Autodesk Fusion 360 part; units mm, degrees
(part 2 of 3)
  line L1095 (-31.3966, -14.5) -> (-31.3966, -13.5)
  line L1096 (26.2931, -7) -> (27.2931, -7)
  line L1097 (-33.9483, -11) -> (-34.9483, -11)
  line L1098 (-31.3966, -11) -> (-32.3966, -11)
  line L1099 (-27.2931, -11) -> (-27.2931, -12)
  line L1100 (-28.8448, -12) -> (-28.8448, -11)
  line L1101 (-34.9483, -14.5) -> (-33.9483, -14.5)
  line L1102 (-33.9483, -13.5) -> (-34.9483, -13.5)
  line L1103 (-34.9483, -13.5) -> (-34.9483, -14.5)
  line L1104 (-31.5, -23) -> (-30.5, -23)
  line L1105 (-31.5, -21.5) -> (-31.5, -20.5)
  line L1106 (-30.5, -24) -> (-31.5, -24)
  line L1107 (-34, -23) -> (-33, -23)
  line L1108 (-28, -23) -> (-28, -24)
  line L1109 (-33, -20.5) -> (-33, -21.5)
  line L1110 (-36.5, -12) -> (-36.5, -11)
  line L1111 (22.1897, -3.5) -> (21.1897, -3.5)
  line L1112 (21.1897, -7) -> (22.1897, -7)
  line L1113 (-34.9483, -11) -> (-34.9483, -12)
  line L1114 (-29, -24) -> (-29, -23)
  line L1115 (-35.5, -23) -> (-35.5, -24)
  line L1116 (-36.5, -21.5) -> (-36.5, -20.5)
  line L1117 (-33.9483, -14.5) -> (-33.9483, -13.5)
  line L1118 (-29, -23) -> (-28, -23)
  line L1119 (-31.3966, -13.5) -> (-32.3966, -13.5)
  line L1120 (-36.5, -23) -> (-35.5, -23)
  line L1121 (-32.3966, -12) -> (-31.3966, -12)
  line L1122 (-33, -21.5) -> (-34, -21.5)
  line L1123 (-27.2931, -13.5) -> (-27.2931, -14.5)
  line L1124 (-29.8448, -12) -> (-28.8448, -12)
  line L1125 (-32.3966, -13.5) -> (-32.3966, -14.5)
  line L1126 (-37.5, -14.5) -> (-36.5, -14.5)
  line L1127 (-36.5, -20.5) -> (-35.5, -20.5)
  line L1128 (-36.5, -14.5) -> (-36.5, -13.5)
  line L1129 (-37.5, -11) -> (-37.5, -12)
  line L1130 (-29, -21.5) -> (-29, -20.5)
  line L1131 (-28.8448, -11) -> (-29.8448, -11)
  line L1132 (-34, -20.5) -> (-33, -20.5)
  line L1133 (-35.5, -20.5) -> (-35.5, -21.5)
  line L1134 (-33.9483, -12) -> (-33.9483, -11)
  line L1135 (-31.5, -24) -> (-31.5, -23)
  line L1136 (-33, -23) -> (-33, -24)
  line L1137 (-36.5, -13.5) -> (-37.5, -13.5)
  line L1138 (-29.8448, -14.5) -> (-28.8448, -14.5)
  line L1139 (36.5, -24) -> (35.5, -24)
  line L1140 (35.5, -20.5) -> (36.5, -20.5)
  line L1141 (36.5, -7) -> (37.5, -7)
  line L1142 (-6.8793, -11) -> (-6.8793, -12)
  line L1143 (-8.431, -12) -> (-8.431, -11)
  line L1144 (5.8793, -8.5) -> (5.8793, -9.5)
  line L1145 (4.3276, -9.5) -> (4.3276, -8.5)
  line L1146 (33.9483, -13.5) -> (33.9483, -14.5)
  line L1147 (3.3276, -8.5) -> (3.3276, -9.5)
  line L1148 (6.8793, -8.5) -> (5.8793, -8.5)
  line L1149 (3.3276, -11) -> (3.3276, -12)
  line L1150 (37.5, -7) -> (37.5, -6)
  line L1151 (1.7759, -8.5) -> (0.7759, -8.5)
  line L1152 (-5.8793, -7) -> (-5.8793, -6)
  line L1153 (-8.431, -3.5) -> (-9.431, -3.5)
  line L1154 (4.3276, -8.5) -> (3.3276, -8.5)
  line L1155 (36.5, -23) -> (35.5, -24) construction
  line L1156 (36.5, -6) -> (36.5, -7)
  line L1157 (5.8793, -12) -> (6.8793, -12)
  line L1158 (34, -23) -> (34, -24)
  line L1159 (0.7759, -9.5) -> (1.7759, -9.5)
  line L1160 (-9.431, -11) -> (-9.431, -12)
  line L1161 (37.5, -6) -> (36.5, -6)
  line L1162 (36.5, -21.5) -> (35.5, -21.5)
  line L1163 (-10.9828, -9.5) -> (-10.9828, -8.5)
  line L1164 (-9.431, -8.5) -> (-9.431, -9.5)
  line L1165 (33.9483, -3.5) -> (33.9483, -4.5)
  line L1166 (0.7759, -11) -> (0.7759, -12)
  line L1167 (-6.8793, -7) -> (-5.8793, -7)
  line L1168 (35.5, -21.5) -> (35.5, -20.5)
  line L1169 (36.5, -4.5) -> (37.5, -3.5) construction
  line L1170 (-5.8793, -4.5) -> (-5.8793, -3.5)
  line L1171 (33.9483, -11) -> (33.9483, -12)
  line L1172 (34.9483, -12) -> (34.9483, -11)
  line L1173 (36.5, -4.5) -> (37.5, -4.5)
  line L1174 (33.9483, -14.5) -> (34.9483, -14.5)
  line L1175 (-9.431, -9.5) -> (-8.431, -9.5)
  line L1176 (37.5, -13.5) -> (36.5, -13.5)
  line L1177 (-6.8793, -8.5) -> (-6.8793, -9.5)
  line L1178 (-8.431, -8.5) -> (-9.431, -8.5)
  line L1179 (-9.431, -12) -> (-8.431, -12)
  line L1180 (36.5, -3.5) -> (36.5, -4.5)
  line L1181 (3.3276, -6) -> (3.3276, -7)
  line L1182 (-9.431, -4.5) -> (-8.431, -4.5)
  line L1183 (-5.8793, -12) -> (-5.8793, -11)
  line L1184 (36.5, -13.5) -> (36.5, -14.5)
  line L1185 (1.7759, -12) -> (1.7759, -11)
  line L1186 (34.9483, -3.5) -> (33.9483, -3.5)
  line L1187 (37.5, -4.5) -> (36.5, -3.5) construction
  line L1188 (-6.8793, -9.5) -> (-5.8793, -9.5)
  line L1189 (-5.8793, -3.5) -> (-6.8793, -3.5)
  line L1190 (34.9483, -13.5) -> (33.9483, -13.5)
  line L1191 (1.7759, -6) -> (0.7759, -6)
  line L1192 (-5.8793, -8.5) -> (-6.8793, -8.5)
  line L1193 (34.9483, -11) -> (33.9483, -11)
  line L1194 (37.5, -3.5) -> (36.5, -3.5)
  line L1195 (37.5, -4.5) -> (37.5, -3.5)
  line L1196 (1.7759, -4.5) -> (1.7759, -3.5)
  line L1197 (36.5, -14.5) -> (37.5, -14.5)
  line L1198 (-8.431, -11) -> (-9.431, -11)
  line L1199 (34.9483, -14.5) -> (34.9483, -13.5)
  line L1200 (3.3276, -9.5) -> (4.3276, -9.5)
  line L1201 (33.9483, -4.5) -> (34.9483, -4.5)
  line L1202 (37.5, -14.5) -> (37.5, -13.5)
  line L1203 (-6.8793, -6) -> (-6.8793, -7)
  line L1204 (34.9483, -4.5) -> (34.9483, -3.5)
  line L1205 (17.5, -24) -> (17.5, -23)
  line L1206 (15, -23) -> (16, -23)
  line L1207 (12.5, -20.5) -> (13.5, -20.5)
  line L1208 (18.5, -23) -> (18.5, -24)
  line L1209 (17.5, -23) -> (18.5, -23)
  line L1210 (-10.9828, -8.5) -> (-11.9828, -8.5)
  line L1211 (-10.9828, -3.5) -> (-11.9828, -3.5)
  line L1212 (-11.9828, -7) -> (-10.9828, -7)
  line L1213 (13.5345, -8.5) -> (13.5345, -9.5)
  line L1214 (19.6379, -8.5) -> (18.6379, -8.5)
  line L1215 (-11.9828, -12) -> (-10.9828, -12)
  line L1216 (-11.9828, -4.5) -> (-10.9828, -4.5)
  line L1217 (-10.9828, -6) -> (-11.9828, -6)
  line L1218 (-11.9828, -14.5) -> (-10.9828, -14.5)
  line L1219 (-15, -24) -> (-16, -24)
  line L1220 (-15, -23) -> (-15, -24)
  line L1221 (15, -20.5) -> (16, -20.5)
  line L1222 (-13.5, -21.5) -> (-13.5, -20.5)
  line L1223 (-14.5345, -8.5) -> (-14.5345, -9.5)
  line L1224 (-11.9828, -6) -> (-11.9828, -7)
  line L1225 (-16.0862, -8.5) -> (-17.0862, -8.5)
  line L1226 (-17.0862, -14.5) -> (-16.0862, -14.5)
  line L1227 (14.5345, -14.5) -> (14.5345, -13.5)
  line L1228 (14.5345, -13.5) -> (13.5345, -13.5)
  line L1229 (19.6379, -14.5) -> (19.6379, -13.5)
  line L1230 (14.5345, -11) -> (13.5345, -11)
  line L1231 (17.0862, -12) -> (17.0862, -11)
  line L1232 (-16.0862, -3.5) -> (-17.0862, -3.5)
  line L1233 (-13.5345, -4.5) -> (-13.5345, -3.5)
  line L1234 (-13.5345, -14.5) -> (-13.5345, -13.5)
  line L1235 (13.5345, -12) -> (14.5345, -12)
  line L1236 (19.6379, -12) -> (19.6379, -11)
  line L1237 (-13.5345, -8.5) -> (-14.5345, -8.5)
  line L1238 (-14.5345, -9.5) -> (-13.5345, -9.5)
  line L1239 (-14.5345, -3.5) -> (-14.5345, -4.5)
  line L1240 (-14.5345, -6) -> (-14.5345, -7)
  line L1241 (14.5345, -12) -> (14.5345, -11)
  line L1242 (-14.5345, -14.5) -> (-13.5345, -14.5)
  line L1243 (17.0862, -13.5) -> (16.0862, -13.5)
  line L1244 (16.0862, -14.5) -> (17.0862, -14.5)
  line L1245 (-14.5345, -4.5) -> (-13.5345, -4.5)
  line L1246 (18.6379, -13.5) -> (18.6379, -14.5)
  line L1247 (-14.5345, -12) -> (-13.5345, -12)
  line L1248 (17.0862, -14.5) -> (17.0862, -13.5)
  line L1249 (-20, -20.5) -> (-20, -21.5)
  line L1250 (-27.2931, -14.5) -> (-26.2931, -14.5)
  line L1251 (-18.5, -21.5) -> (-18.5, -20.5)
  line L1252 (22.1897, -11) -> (21.1897, -11)
  line L1253 (19.6379, -9.5) -> (19.6379, -8.5)
  line L1254 (17.0862, -3.5) -> (16.0862, -3.5)
  line L1255 (14.5345, -7) -> (14.5345, -6)
  line L1256 (21, -23) -> (20, -24) construction
  line L1257 (-21, -24) -> (-21, -23)
  line L1258 (-17.5, -24) -> (-18.5, -24)
  line L1259 (-18.5, -20.5) -> (-17.5, -20.5)
  line L1260 (-18.5, -23) -> (-17.5, -23)
  line L1261 (18.6379, -7) -> (19.6379, -7)
  line L1262 (16.0862, -6) -> (16.0862, -7)
  line L1263 (14.5345, -3.5) -> (13.5345, -3.5)
  line L1264 (-26.5, -23) -> (-25.5, -24) construction
  line L1265 (13.5345, -9.5) -> (14.5345, -9.5)
  line L1266 (-16.0862, -6) -> (-17.0862, -6)
  line L1267 (-26.5, -23) -> (-25.5, -23)
  line L1268 (-20, -23) -> (-20, -24)
  line L1269 (18.6379, -4.5) -> (19.6379, -4.5)
  line L1270 (-25.5, -24) -> (-26.5, -24)
  line L1271 (-26.2931, -11) -> (-27.2931, -11)
  line L1272 (16.0862, -8.5) -> (16.0862, -9.5)
  line L1273 (-26.5, -24) -> (-26.5, -23)
  line L1274 (14.5345, -9.5) -> (14.5345, -8.5)
  line L1275 (-20, -24) -> (-21, -24)
  line L1276 (21, -24) -> (20, -24)
  line L1277 (-21, -23) -> (-20, -23)
  line L1278 (17.0862, -7) -> (17.0862, -6)
  line L1279 (13.5345, -6) -> (13.5345, -7)
  line L1280 (19.6379, -4.5) -> (19.6379, -3.5)
  line L1281 (17.0862, -9.5) -> (17.0862, -8.5)
  line L1282 (13.5345, -3.5) -> (13.5345, -4.5)
  line L1283 (14.5345, -8.5) -> (13.5345, -8.5)
  line L1284 (20, -23) -> (21, -24) construction
  line L1285 (-25.5, -23) -> (-25.5, -24)
  line L1286 (18.6379, -9.5) -> (19.6379, -9.5)
  line L1287 (16.0862, -3.5) -> (16.0862, -4.5)
  line L1288 (-17.0862, -7) -> (-16.0862, -7)
  line L1289 (16.0862, -4.5) -> (17.0862, -4.5)
  line L1290 (-26.5, -21.5) -> (-26.5, -20.5)
  line L1291 (21, -21.5) -> (20, -21.5)
  line L1292 (16.0862, -9.5) -> (17.0862, -9.5)
  line L1293 (16.0862, -7) -> (17.0862, -7)
  line L1294 (17.0862, -6) -> (16.0862, -6)
  line L1295 (-16.0862, -13.5) -> (-17.0862, -13.5)
  line L1296 (19.6379, -6) -> (18.6379, -6)
  line L1297 (18.6379, -3.5) -> (18.6379, -4.5)
  line L1298 (-37.5, -7) -> (-36.5, -7)
  line L1299 (-33.9483, -9.5) -> (-33.9483, -8.5)
  line L1300 (-24.7414, -13.5) -> (-24.7414, -14.5)
  line L1301 (-23.7414, -12) -> (-23.7414, -11)
  line L1302 (-28.8448, -4.5) -> (-28.8448, -3.5)
  line L1303 (-22.1897, -11) -> (-22.1897, -12)
  line L1304 (-18.6379, -7) -> (-18.6379, -6)
  line L1305 (-33.9483, -6) -> (-34.9483, -6)
  line L1306 (-26.2931, -13.5) -> (-27.2931, -13.5)
  line L1307 (-36.5, -6) -> (-37.5, -6)
  line L1308 (-19.6379, -12) -> (-18.6379, -12)
  line L1309 (-26.2931, -3.5) -> (-27.2931, -3.5)
  line L1310 (-27.2931, -6) -> (-27.2931, -7)
  line L1311 (23.7414, -11) -> (23.7414, -12)
  line L1312 (-21.1897, -4.5) -> (-21.1897, -3.5)
  line L1313 (21.1897, -3.5) -> (21.1897, -4.5)
  line L1314 (-28.8448, -6) -> (-29.8448, -6)
  line L1315 (-32.3966, -6) -> (-32.3966, -7)
  line L1316 (-23.7414, -8.5) -> (-24.7414, -8.5)
  line L1317 (-33.9483, -7) -> (-33.9483, -6)
  line L1318 (-34.9483, -4.5) -> (-33.9483, -4.5)
  line L1319 (-27.2931, -9.5) -> (-26.2931, -9.5)
  line L1320 (-26.2931, -9.5) -> (-26.2931, -8.5)
  line L1321 (-27.2931, -3.5) -> (-27.2931, -4.5)
  line L1322 (-31.3966, -7) -> (-31.3966, -6)
  line L1323 (23.7414, -8.5) -> (23.7414, -9.5)
  line L1324 (-24.7414, -8.5) -> (-24.7414, -9.5)
  line L1325 (-26.2931, -14.5) -> (-26.2931, -13.5)
  line L1326 (-22.1897, -13.5) -> (-22.1897, -14.5)
  line L1327 (27.2931, -3.5) -> (26.2931, -3.5)
  line L1328 (-34.9483, -9.5) -> (-33.9483, -9.5)
  line L1329 (-29.8448, -4.5) -> (-28.8448, -4.5)
  line L1330 (-18.6379, -12) -> (-18.6379, -11)
  line L1331 (-37.5, -6) -> (-37.5, -7)
  line L1332 (-24.7414, -9.5) -> (-23.7414, -9.5)
  line L1333 (-31.3966, -12) -> (-31.3966, -11)
  line L1334 (-26.2931, -6) -> (-27.2931, -6)
  line L1335 (-17.0862, -13.5) -> (-17.0862, -14.5)
  line L1336 (-22.1897, -14.5) -> (-21.1897, -14.5)
  line L1337 (-23.7414, -9.5) -> (-23.7414, -8.5)
  line L1338 (-37.5, -3.5) -> (-37.5, -4.5)
  line L1339 (-27.2931, -12) -> (-26.2931, -12)
  line L1340 (-18.6379, -8.5) -> (-19.6379, -8.5)
  line L1341 (-24.7414, -4.5) -> (-23.7414, -4.5)
  line L1342 (-19.6379, -7) -> (-18.6379, -7)
  line L1343 (-21.1897, -9.5) -> (-21.1897, -8.5)
  line L1344 (-21.1897, -8.5) -> (-22.1897, -8.5)
  line L1345 (-31.3966, -9.5) -> (-31.3966, -8.5)
  line L1346 (-37.5, -9.5) -> (-36.5, -9.5)
  line L1347 (27.2931, -7) -> (27.2931, -6)
  line L1348 (-23.7414, -3.5) -> (-24.7414, -3.5)
  line L1349 (-31.3966, -4.5) -> (-31.3966, -3.5)
  line L1350 (-18.6379, -6) -> (-19.6379, -6)
  line L1351 (-18.6379, -13.5) -> (-19.6379, -13.5)
  line L1352 (-33.9483, -8.5) -> (-34.9483, -8.5)
  line L1353 (-21.1897, -7) -> (-21.1897, -6)
  line L1354 (-37.5, -8.5) -> (-37.5, -9.5)
  line L1355 (-34.9483, -7) -> (-33.9483, -7)
  line L1356 (-22.1897, -12) -> (-21.1897, -12)
  line L1357 (-27.2931, -7) -> (-26.2931, -7)
  line L1358 (-29.8448, -11) -> (-29.8448, -12)
  line L1359 (-17.0862, -11) -> (-17.0862, -12)
  line L1360 (-24.7414, -14.5) -> (-23.7414, -14.5)
  line L1361 (22.1897, -7) -> (22.1897, -6)
  line L1362 (-32.3966, -14.5) -> (-31.3966, -14.5)
  line L1363 (-19.6379, -14.5) -> (-18.6379, -14.5)
  line L1364 (-37.5, -13.5) -> (-37.5, -14.5)
  line L1365 (-23.7414, -13.5) -> (-24.7414, -13.5)
  line L1366 (-33, -24) -> (-34, -24)
  line L1367 (-21.1897, -11) -> (-22.1897, -11)
  line L1368 (-27.2931, -8.5) -> (-27.2931, -9.5)
  line L1369 (-30.5, -21.5) -> (-31.5, -21.5)
  line L1370 (-24.7414, -7) -> (-23.7414, -7)
  line L1371 (23.7414, -3.5) -> (23.7414, -4.5)
  line L1372 (23.7414, -7) -> (24.7414, -7)
  line L1373 (26.2931, -3.5) -> (26.2931, -4.5)
  line L1374 (-26.2931, -12) -> (-26.2931, -11)
  line L1375 (21.1897, -4.5) -> (22.1897, -4.5)
  line L1376 (-21.1897, -12) -> (-21.1897, -11)
  line L1377 (-34, -21.5) -> (-34, -20.5)
  line L1378 (-28, -20.5) -> (-28, -21.5)
  line L1379 (-28, -24) -> (-29, -24)
  line L1380 (-29, -20.5) -> (-28, -20.5)
  line L1381 (24.7414, -7) -> (24.7414, -6)
  line L1382 (-27.2931, -4.5) -> (-26.2931, -4.5)
  line L1383 (-28.8448, -14.5) -> (-28.8448, -13.5)
  line L1384 (-35.5, -21.5) -> (-36.5, -21.5)
  line L1385 (-24.7414, -11) -> (-24.7414, -12)
  line L1386 (21.1897, -6) -> (21.1897, -7)
  line L1387 (-30.5, -23) -> (-30.5, -24)
  line L1388 (-23.7414, -11) -> (-24.7414, -11)
  line L1389 (26.2931, -4.5) -> (27.2931, -4.5)
  line L1390 (-19.6379, -11) -> (-19.6379, -12)
  line L1391 (-34, -24) -> (-34, -23)
  line L1392 (-23.7414, -4.5) -> (-23.7414, -3.5)
  line L1393 (-32.3966, -11) -> (-32.3966, -12)
  line L1394 (27.2931, -6) -> (26.2931, -6)
  line L1395 (-23.7414, -6) -> (-24.7414, -6)
  line L1396 (-21.1897, -14.5) -> (-21.1897, -13.5)
  line L1397 (24.7414, -4.5) -> (24.7414, -3.5)
  line L1398 (26.2931, -6) -> (26.2931, -7)
  line L1399 (22.1897, -4.5) -> (22.1897, -3.5)
  line L1400 (-23.7414, -14.5) -> (-23.7414, -13.5)
  line L1401 (-31.5, -20.5) -> (-30.5, -20.5)
  line L1402 (23.7414, -4.5) -> (24.7414, -4.5)
  line L1403 (23.7414, -6) -> (23.7414, -7)
  line L1404 (27.2931, -4.5) -> (27.2931, -3.5)
  line L1405 (22.1897, -6) -> (21.1897, -6)
  line L1406 (-24.7414, -12) -> (-23.7414, -12)
  line L1407 (-18.6379, -14.5) -> (-18.6379, -13.5)
  line L1408 (-35.5, -24) -> (-36.5, -24)
  line L1409 (-30.5, -20.5) -> (-30.5, -21.5)
  line L1410 (24.7414, -6) -> (23.7414, -6)
  line L1411 (-29.8448, -13.5) -> (-29.8448, -14.5)
  line L1412 (-34.9483, -12) -> (-33.9483, -12)
  line L1413 (-36.5, -24) -> (-36.5, -23)
  line L1414 (-16.0862, -12) -> (-16.0862, -11)
  line L1415 (20, -20.5) -> (21, -20.5)
  line L1416 (-11.9828, -11) -> (-11.9828, -12)
  line L1417 (-13.5345, -3.5) -> (-14.5345, -3.5)
  line L1418 (-16.0862, -4.5) -> (-16.0862, -3.5)
  line L1419 (-14.5345, -13.5) -> (-14.5345, -14.5)
  line L1420 (-13.5345, -12) -> (-13.5345, -11)
  line L1421 (-16.0862, -11) -> (-17.0862, -11)
  line L1422 (-13.5345, -7) -> (-13.5345, -6)
  line L1423 (13.5, -24) -> (12.5, -24)
  line L1424 (-13.5345, -11) -> (-14.5345, -11)
  line L1425 (-11.9828, -13.5) -> (-11.9828, -14.5)
  line L1426 (16.0862, -13.5) -> (16.0862, -14.5)
  line L1427 (18.6379, -14.5) -> (19.6379, -14.5)
  line L1428 (-16.0862, -9.5) -> (-16.0862, -8.5)
  line L1429 (13.5345, -14.5) -> (14.5345, -14.5)
  line L1430 (17.0862, -11) -> (16.0862, -11)
  line L1431 (-17.0862, -12) -> (-16.0862, -12)
  line L1432 (18.6379, -11) -> (18.6379, -12)
  line L1433 (18.6379, -8.5) -> (18.6379, -9.5)
  line L1434 (-18.6379, -9.5) -> (-18.6379, -8.5)
  line L1435 (-31.3966, -8.5) -> (-32.3966, -8.5)
  line L1436 (-32.3966, -9.5) -> (-31.3966, -9.5)
  line L1437 (23.7414, -9.5) -> (24.7414, -9.5)
  line L1438 (25.5, -21.5) -> (25.5, -20.5)
  line L1439 (21.1897, -13.5) -> (21.1897, -14.5)
  line L1440 (22.1897, -13.5) -> (21.1897, -13.5)
  line L1441 (-25.5, -23) -> (-26.5, -24) construction
  line L1442 (18.6379, -6) -> (18.6379, -7)
  line L1443 (-29.8448, -8.5) -> (-29.8448, -9.5)
  line L1444 (-20, -21.5) -> (-21, -21.5)
  line L1445 (26.2931, -9.5) -> (27.2931, -9.5)
  line L1446 (-17.5, -21.5) -> (-18.5, -21.5)
  line L1447 (-18.6379, -4.5) -> (-18.6379, -3.5)
  line L1448 (21.1897, -11) -> (21.1897, -12)
  line L1449 (24.7414, -12) -> (24.7414, -11)
  line L1450 (-31.3966, -6) -> (-32.3966, -6)
  line L1451 (-26.5, -20.5) -> (-25.5, -20.5)
  line L1452 (-17.5, -23) -> (-17.5, -24)
  line L1453 (-17.0862, -3.5) -> (-17.0862, -4.5)
  line L1454 (-19.6379, -6) -> (-19.6379, -7)
  line L1455 (27.2931, -9.5) -> (27.2931, -8.5)
  line L1456 (26.5, -23) -> (26.5, -24)
  line L1457 (-32.3966, -3.5) -> (-32.3966, -4.5)
  line L1458 (17.0862, -4.5) -> (17.0862, -3.5)
  line L1459 (-21, -20.5) -> (-20, -20.5)
  line L1460 (23.7414, -14.5) -> (24.7414, -14.5)
  line L1461 (24.7414, -8.5) -> (23.7414, -8.5)
  line L1462 (26.2931, -11) -> (26.2931, -12)
  line L1463 (14.5345, -6) -> (13.5345, -6)
  line L1464 (24.7414, -9.5) -> (24.7414, -8.5)
  line L1465 (-25.5, -21.5) -> (-26.5, -21.5)
  line L1466 (-22.1897, -4.5) -> (-21.1897, -4.5)
  line L1467 (14.5345, -4.5) -> (14.5345, -3.5)
  line L1468 (21, -20.5) -> (21, -21.5)
  line L1469 (24.7414, -14.5) -> (24.7414, -13.5)
  line L1470 (21.1897, -12) -> (22.1897, -12)
  line L1471 (13.5345, -4.5) -> (14.5345, -4.5)
  line L1472 (-25.5, -20.5) -> (-25.5, -21.5)
  line L1473 (22.1897, -9.5) -> (22.1897, -8.5)
  line L1474 (17.0862, -8.5) -> (16.0862, -8.5)
  line L1475 (19.6379, -7) -> (19.6379, -6)
  line L1476 (24.7414, -13.5) -> (23.7414, -13.5)
  line L1477 (21, -23) -> (21, -24)
  line L1478 (25.5, -20.5) -> (26.5, -20.5)
  line L1479 (-18.5, -24) -> (-18.5, -23)
  line L1480 (-22.1897, -9.5) -> (-21.1897, -9.5)
  line L1481 (13.5345, -7) -> (14.5345, -7)
  line L1482 (-31.3966, -3.5) -> (-32.3966, -3.5)
  line L1483 (21.1897, -9.5) -> (22.1897, -9.5)
  line L1484 (27.2931, -8.5) -> (26.2931, -8.5)
  line L1485 (27.2931, -13.5) -> (26.2931, -13.5)
  line L1486 (26.2931, -13.5) -> (26.2931, -14.5)
  line L1487 (-17.5, -20.5) -> (-17.5, -21.5)
  line L1488 (21.1897, -14.5) -> (22.1897, -14.5)
  line L1489 (-21, -21.5) -> (-21, -20.5)
  line L1490 (19.6379, -3.5) -> (18.6379, -3.5)
  line L1491 (-29.8448, -7) -> (-28.8448, -7)
  line L1492 (-19.6379, -4.5) -> (-18.6379, -4.5)
  line L1493 (27.2931, -14.5) -> (27.2931, -13.5)
  line L1494 (-19.6379, -9.5) -> (-18.6379, -9.5)
  line L1495 (-34.9483, -8.5) -> (-34.9483, -9.5)
  line L1496 (-28.8448, -8.5) -> (-29.8448, -8.5)
  line L1497 (-33.9483, -3.5) -> (-34.9483, -3.5)
  line L1498 (26.2931, -14.5) -> (27.2931, -14.5)
  line L1499 (-36.5, -4.5) -> (-36.5, -3.5)
  line L1500 (22.1897, -8.5) -> (21.1897, -8.5)
  line L1501 (-33.9483, -4.5) -> (-33.9483, -3.5)
  line L1502 (-19.6379, -3.5) -> (-19.6379, -4.5)
  line L1503 (-32.3966, -4.5) -> (-31.3966, -4.5)
  line L1504 (-36.5, -9.5) -> (-36.5, -8.5)
  line L1505 (-29.8448, -9.5) -> (-28.8448, -9.5)
  line L1506 (23.7414, -12) -> (24.7414, -12)
  line L1507 (-32.3966, -7) -> (-31.3966, -7)
  line L1508 (-34.9483, -3.5) -> (-34.9483, -4.5)
  line L1509 (-28.8448, -3.5) -> (-29.8448, -3.5)
  line L1510 (-23.7414, -7) -> (-23.7414, -6)
  line L1511 (22.1897, -12) -> (22.1897, -11)
  line L1512 (-21.1897, -6) -> (-22.1897, -6)
  line L1513 (-36.5, -7) -> (-36.5, -6)
  line L1514 (-18.6379, -3.5) -> (-19.6379, -3.5)
  line L1515 (-29.8448, -3.5) -> (-29.8448, -4.5)
  line L1516 (-32.3966, -8.5) -> (-32.3966, -9.5)
  line L1517 (27.2931, -12) -> (27.2931, -11)
  line L1518 (-36.5, -8.5) -> (-37.5, -8.5)
  line L1519 (21.1897, -8.5) -> (21.1897, -9.5)
  line L1520 (25.5, -24) -> (25.5, -23)
  line L1521 (-34.9483, -6) -> (-34.9483, -7)
  line L1522 (26.2931, -8.5) -> (26.2931, -9.5)
  line L1523 (26.2931, -12) -> (27.2931, -12)
  line L1524 (-26.2931, -4.5) -> (-26.2931, -3.5)
  line L1525 (-19.6379, -13.5) -> (-19.6379, -14.5)
  line L1526 (-19.6379, -8.5) -> (-19.6379, -9.5)
  line L1527 (-22.1897, -8.5) -> (-22.1897, -9.5)
  line L1528 (27.2931, -11) -> (26.2931, -11)
  line L1529 (25.5, -23) -> (26.5, -23)
  line L1530 (26.5, -21.5) -> (25.5, -21.5)
  line L1531 (-22.1897, -7) -> (-21.1897, -7)
  line L1532 (-26.2931, -8.5) -> (-27.2931, -8.5)
  line L1533 (-37.5, -4.5) -> (-36.5, -4.5)
  line L1534 (-17.0862, -6) -> (-17.0862, -7)
  line L1535 (26.5, -24) -> (25.5, -24)
  line L1536 (24.7414, -11) -> (23.7414, -11)
  line L1537 (-22.1897, -3.5) -> (-22.1897, -4.5)
  line L1538 (26.5, -20.5) -> (26.5, -21.5)
  line L1539 (-28.8448, -9.5) -> (-28.8448, -8.5)
  line L1540 (-24.7414, -6) -> (-24.7414, -7)
  line L1541 (23.7414, -13.5) -> (23.7414, -14.5)
  line L1542 (-17.0862, -8.5) -> (-17.0862, -9.5)
  line L1543 (-24.7414, -3.5) -> (-24.7414, -4.5)
  line L1544 (-22.1897, -6) -> (-22.1897, -7)
  line L1545 (-26.2931, -7) -> (-26.2931, -6)
  line L1546 (-18.6379, -11) -> (-19.6379, -11)
  line L1547 (-36.5, -3.5) -> (-37.5, -3.5)
  line L1548 (-21.1897, -13.5) -> (-22.1897, -13.5)
  line L1549 (22.1897, -14.5) -> (22.1897, -13.5)
  line L1550 (-28.8448, -7) -> (-28.8448, -6)
  line L1551 (-29.8448, -6) -> (-29.8448, -7)
  line L1552 (-21.1897, -3.5) -> (-22.1897, -3.5)
  line L1553 (28.8448, -7) -> (29.8448, -7)
  line L1554 (29.8448, -13.5) -> (28.8448, -13.5)
  line L1555 (28.8448, -13.5) -> (28.8448, -14.5)
  line L1556 (4.5, -23) -> (5.5, -24) construction
  line L1557 (29.8448, -7) -> (29.8448, -6)
  line L1558 (-6.8793, -13.5) -> (-6.8793, -14.5)
  line L1559 (29.8448, -14.5) -> (29.8448, -13.5)
  line L1560 (-8.431, -14.5) -> (-8.431, -13.5)
  line L1561 (3, -24) -> (2, -24)
  line L1562 (-9.431, -13.5) -> (-9.431, -14.5)
  line L1563 (6.8793, -14.5) -> (6.8793, -13.5)
  line L1564 (5.5, -23) -> (5.5, -24)
  line L1565 (29.8448, -6) -> (28.8448, -6)
  line L1566 (3, -20.5) -> (3, -21.5)
  line L1567 (-10.9828, -14.5) -> (-10.9828, -13.5)
  line L1568 (-10, -21.5) -> (-11, -21.5)
  line L1569 (3.3276, -14.5) -> (4.3276, -14.5)
  line L1570 (-0.7759, -11) -> (-1.7759, -11)
  line L1571 (-1.7759, -12) -> (-0.7759, -12)
  line L1572 (11.9828, -11) -> (10.9828, -11)
  line L1573 (-3.3276, -6) -> (-4.3276, -6)
  line L1574 (-0.7759, -13.5) -> (-1.7759, -13.5)
  line L1575 (8.431, -3.5) -> (8.431, -4.5)
  line L1576 (-0.7759, -14.5) -> (-0.7759, -13.5)
  line L1577 (8.431, -9.5) -> (9.431, -9.5)
  line L1578 (10.9828, -11) -> (10.9828, -12)
  line L1579 (-1.7759, -11) -> (-1.7759, -12)
  line L1580 (9.431, -11) -> (8.431, -11)
  line L1581 (-4.3276, -3.5) -> (-4.3276, -4.5)
  line L1582 (8.431, -7) -> (9.431, -7)
  line L1583 (-4.3276, -6) -> (-4.3276, -7)
  line L1584 (-3.3276, -7) -> (-3.3276, -6)
  line L1585 (-1.7759, -6) -> (-1.7759, -7)
  line L1586 (9.431, -7) -> (9.431, -6)
  line L1587 (-1.7759, -7) -> (-0.7759, -7)
  line L1588 (-3.3276, -3.5) -> (-4.3276, -3.5)
  line L1589 (10.9828, -7) -> (11.9828, -7)
  line L1590 (10.9828, -4.5) -> (11.9828, -4.5)
  line L1591 (-4.3276, -8.5) -> (-4.3276, -9.5)
  line L1592 (10.9828, -3.5) -> (10.9828, -4.5)
  line L1593 (11.9828, -8.5) -> (10.9828, -8.5)
  line L1594 (-3.3276, -8.5) -> (-4.3276, -8.5)
  line L1595 (11.9828, -7) -> (11.9828, -6)
  line L1596 (9.431, -4.5) -> (9.431, -3.5)
  line L1597 (-1.7759, -9.5) -> (-0.7759, -9.5)
  line L1598 (-1.7759, -8.5) -> (-1.7759, -9.5)
  line L1599 (9.431, -9.5) -> (9.431, -8.5)
  line L1600 (-1.7759, -3.5) -> (-1.7759, -4.5)
  line L1601 (10, -23) -> (11, -23)
  line L1602 (12.5, -21.5) -> (12.5, -20.5)
  line L1603 (-3, -21.5) -> (-3, -20.5)
  line L1604 (-2, -21.5) -> (-3, -21.5)
  line L1605 (11, -23) -> (11, -24)
  line L1606 (-2, -20.5) -> (-2, -21.5)
  line L1607 (-4.5, -23) -> (-4.5, -24)
  line L1608 (-0.5, -23) -> (0.5, -23)
  line L1609 (10, -20.5) -> (11, -20.5)
  line L1610 (10, -24) -> (10, -23)
  line L1611 (10.9828, -13.5) -> (10.9828, -14.5)
  line L1612 (9.431, -14.5) -> (9.431, -13.5)
  line L1613 (9.431, -13.5) -> (8.431, -13.5)
  line L1614 (11, -21.5) -> (10, -21.5)
  line L1615 (11.9828, -14.5) -> (11.9828, -13.5)
  line L1616 (-1.7759, -13.5) -> (-1.7759, -14.5)
  line L1617 (10.9828, -14.5) -> (11.9828, -14.5)
  line L1618 (-1.7759, -14.5) -> (-0.7759, -14.5)
  line L1619 (10, -21.5) -> (10, -20.5)
  line L1620 (-3.3276, -11) -> (-4.3276, -11)
  line L1621 (-3.3276, -13.5) -> (-4.3276, -13.5)
  line L1622 (8.431, -13.5) -> (8.431, -14.5)
  line L1623 (11, -24) -> (10, -24)
  line L1624 (8.431, -14.5) -> (9.431, -14.5)
  line L1625 (12.5, -24) -> (12.5, -23)
  line L1626 (-4.3276, -11) -> (-4.3276, -12)
  line L1627 (11, -20.5) -> (11, -21.5)
  line L1628 (-3.3276, -12) -> (-3.3276, -11)
  line L1629 (11.9828, -13.5) -> (10.9828, -13.5)
  line L1630 (-4.3276, -14.5) -> (-3.3276, -14.5)
  line L1631 (-3.3276, -14.5) -> (-3.3276, -13.5)
  line L1632 (-4.3276, -13.5) -> (-4.3276, -14.5)
  line L1633 (-4.3276, -12) -> (-3.3276, -12)
  line L1634 (-0.7759, -12) -> (-0.7759, -11)
  point P0 (36, 23.5)
  point P1 (20.5, 23.5)
  point P2 (5, 23.5)
  point P3 (-10.5, 23.5)
  point P4 (-26, 23.5)
  point P5 (37, 4)
  point P6 (36, -23.5)
  point P7 (37, -4)
  point P8 (-26, -23.5)
  point P9 (20.5, -23.5)
  point P10 (5, -23.5)
  point P11 (-10.5, -23.5)
  dimension "d12" = 2
  dimension "d14" = 1
  dimension "d15" = 3
  dimension "d16" = 5
  dimension "d23" = 1
  dimension "d27" = -10
  dimension "d31" = -62
  dimension "d32" = 0
  dimension "d33" = 1
  dimension "d34" = 1
  dimension "d35" = 3
  dimension "d36" = 4
  dimension "d39" = -74
  dimension "d40" = 10
  constraint horizontal L4
  constraint perpendicular L4 L5
  constraint parallel L4 L6
  constraint parallel L5 L7
  constraint coincident L8 origin
  constraint coincident L9 origin
  constraint coincident L0 L4.start
  constraint horizontal L10
  constraint perpendicular L10 L11
  constraint parallel L10 L12
  constraint parallel L11 L13
  constraint coincident L14 P0
  constraint coincident L15 P0
  constraint horizontal L220
  constraint perpendicular L220 L221
  constraint parallel L220 L222
  constraint parallel L221 L223
  constraint coincident L224 P5
  constraint coincident L225 P5
  constraint perpendicular L2 L822
  constraint symmetric L10.start L822 L908.end
  constraint symmetric L10.end L822 L912.end
  constraint symmetric L11.end L822 L929.end
  constraint symmetric L12.end L822 L908.start
  constraint symmetric P0 L822 P6
  constraint symmetric L16.start L822 L982.end
  constraint symmetric L16.end L822 L1008.start
  constraint symmetric L17.end L822 L1008.end
  constraint symmetric L18.end L822 L982.start
  constraint symmetric L20.start L822 L864.start
  constraint symmetric L20.end L822 L863.start
  constraint symmetric L21.end L822 L863.end
  constraint symmetric L22.end L822 L951.end
  constraint symmetric L24.start L822 L939.start
  constraint symmetric L24.end L822 L939.end
  constraint symmetric L25.end L822 L891.start
  constraint symmetric L26.end L822 L891.end
  constraint symmetric L28.start L822 L1520.start
  constraint symmetric L28.end L822 L1520.end
  constraint symmetric L29.end L822 L1456.start
  constraint symmetric L30.end L822 L1456.end
  constraint symmetric L32.start L822 L1162.end
  constraint symmetric L32.end L822 L1140.start
  constraint symmetric L33.end L822 L937.start
  constraint symmetric L34.end L822 L937.end
  constraint symmetric L36.start L822 L975.end
  constraint symmetric L36.end L822 L1007.end
  constraint symmetric L37.end L822 L906.start
  constraint symmetric L38.end L822 L906.end
  constraint symmetric L40.start L822 L947.end
  constraint symmetric L40.end L822 L952.start
  constraint symmetric L41.end L822 L892.start
  constraint symmetric L42.end L822 L892.end
  constraint symmetric L44.start L822 L889.start
  constraint symmetric L44.end L822 L889.end
  constraint symmetric L45.end L822 L888.start
  constraint symmetric L46.end L822 L888.end
  constraint symmetric L48.start L822 L1438.start
  constraint symmetric L48.end L822 L1438.end
  constraint symmetric L49.end L822 L1478.end
  constraint symmetric L50.end L822 L1530.start
  constraint symmetric L52.start L822 L1205.end
  constraint symmetric L52.end L822 L1208.start
  constraint symmetric L53.start L822 L1423.end
  constraint symmetric L53.end L822 L890.start
  constraint symmetric L54.start L822 L896.end
  constraint symmetric L54.end L822 L1081.end
  constraint symmetric L55.start L822 L826.start
  constraint symmetric L55.end L822 L826.end
  constraint symmetric L65.end L822 L823.end
  constraint symmetric L56.start L822 L890.end
  constraint symmetric L56.end L822 L899.end
  constraint symmetric L76.start L822 L1601.end
  constraint symmetric L57.start L822 L1041.end
  constraint symmetric L57.end L822 L1207.start
  constraint symmetric L70.end L822 L1027.end
  constraint symmetric L66.start L822 L1031.end
  constraint symmetric L58.end L822 L1276.start
  constraint symmetric L65.start L822 L823.start
  constraint symmetric L76.end L822 L1605.end
  constraint symmetric L77.end L822 L1610.start
  constraint symmetric L60.start L822 L828.end
  constraint symmetric L60.end L822 L1415.end
  constraint symmetric L72.end L822 L828.start
  constraint symmetric L61.end L822 L896.start
  constraint symmetric L62.end L822 L902.start
  constraint symmetric L80.start L822 L1609.end
  constraint symmetric L64.end L822 L825.start
  constraint symmetric L79.start L822 L1614.start
  constraint symmetric L67.start L822 L831.start
  constraint symmetric L67.end L822 L827.start
  constraint symmetric L68.end L822 L1028.end
  constraint symmetric L82.end L822 L902.end
  constraint symmetric L71.start L822 L825.end
  constraint symmetric L72.start L822 L1291.start
  constraint symmetric L78.end L822 L1601.start
  constraint symmetric L75.start L822 L1614.end
  constraint symmetric L75.end L822 L1609.start
  constraint symmetric P1 L822 P9
  constraint symmetric L87.start L822 L827.end
  constraint symmetric L87.end L822 L829.end
  constraint symmetric L83.end L822 L900.start
  constraint symmetric L94.start L822 L873.end
  constraint symmetric L94.end L822 L852.start
  constraint symmetric L95.start L822 L979.end
  constraint symmetric L95.end L822 L985.end
  constraint symmetric L96.start L822 L887.start
  constraint symmetric L96.end L822 L887.end
  constraint symmetric L97.start L822 L977.start
  constraint symmetric L97.end L822 L977.end
  constraint symmetric L107.end L822 L978.end
  constraint symmetric L98.start L822 L976.start
  constraint symmetric L98.end L822 L976.end
  constraint symmetric L118.start L822 L1037.end
  constraint symmetric L99.start L822 L1603.start
  constraint symmetric L99.end L822 L988.start
  constraint symmetric L112.end L822 L980.start
  constraint symmetric L108.start L822 L980.end
  constraint symmetric L100.end L822 L970.start
  constraint symmetric L107.start L822 L978.start
  constraint symmetric L118.end L822 L1042.start
  constraint symmetric L119.end L822 L960.start
  constraint symmetric L102.start L822 L841.end
  constraint symmetric L102.end L822 L851.end
  constraint symmetric L114.end L822 L841.start
  constraint symmetric L103.end L822 L938.end
  constraint symmetric L104.end L822 L852.end
  constraint symmetric L122.start L822 L984.start
  constraint symmetric L106.end L822 L988.end
  constraint symmetric L121.start L822 L984.end
  constraint symmetric L109.start L822 L842.end
  constraint symmetric L109.end L822 L861.start
  constraint symmetric L110.end L822 L986.end
  constraint symmetric L124.end L822 L873.start
  constraint symmetric L113.start L822 L1604.start
  constraint symmetric L114.start L822 L964.start
  constraint symmetric L120.end L822 L960.end
  constraint symmetric L117.start L822 L962.start
  constraint symmetric L117.end L822 L962.end
  constraint symmetric P2 L822 P10
  constraint symmetric L129.start L822 L861.end
  constraint symmetric L129.end L822 L842.start
  constraint symmetric L125.end L822 L996.end
  constraint symmetric L136.start L822 L832.end
  constraint symmetric L136.end L822 L897.start
  constraint symmetric L137.start L822 L1258.end
  constraint symmetric L137.end L822 L1260.start
  constraint symmetric L138.start L822 L876.end
  constraint symmetric L138.end L822 L959.start
  constraint symmetric L139.start L822 L1026.end
  constraint symmetric L139.end L822 L1023.start
  constraint symmetric L149.end L822 L1219.start
  constraint symmetric L140.start L822 L1260.end
  constraint symmetric L140.end L822 L1258.start
  constraint symmetric L160.start L822 L1268.start
  constraint symmetric L141.start L822 L1251.start
  constraint symmetric L141.end L822 L1251.end
  constraint symmetric L154.end L822 L893.start
  constraint symmetric L150.start L822 L893.end
  constraint symmetric L142.end L822 L877.start
  constraint symmetric L149.start L822 L1048.end
  constraint symmetric L160.end L822 L1268.end
  constraint symmetric L161.end L822 L1257.start
  constraint symmetric L144.start L822 L948.start
  constraint symmetric L144.end L822 L867.start
  constraint symmetric L156.end L822 L1025.start
  constraint symmetric L145.end L822 L876.start
  constraint symmetric L146.end L822 L897.end
  constraint symmetric L164.start L822 L1249.start
  constraint symmetric L148.end L822 L1259.end
  constraint symmetric L163.start L822 L1249.end
  constraint symmetric L151.start L822 L894.start
  constraint symmetric L151.end L822 L894.end
  constraint symmetric L152.end L822 L830.start
  constraint symmetric L166.end L822 L832.start
  constraint symmetric L155.start L822 L1446.start
  constraint symmetric L156.start L822 L867.end
  constraint symmetric L162.end L822 L1257.end
  constraint symmetric L159.start L822 L1444.end
  constraint symmetric L159.end L822 L1459.start
  constraint symmetric P3 L822 P11
  constraint symmetric L171.start L822 L898.end
  constraint symmetric L171.end L822 L895.start
  constraint symmetric L167.end L822 L830.end
  constraint symmetric L178.start L822 L1114.end
  constraint symmetric L178.end L822 L1108.start
  constraint symmetric L179.start L822 L1366.end
  constraint symmetric L179.end L822 L1107.start
  constraint symmetric L180.start L822 L1264.start
  constraint symmetric L180.end L822 L1267.end
  constraint symmetric L181.start L822 L1369.start
  constraint symmetric L181.end L822 L1105.start
  constraint symmetric L191.end L822 L1106.start
  constraint symmetric L182.start L822 L1107.end
  constraint symmetric L182.end L822 L1136.end
  constraint symmetric L202.start L822 L1115.start
  constraint symmetric L183.start L822 L1122.end
  constraint symmetric L183.end L822 L1132.start
  constraint symmetric L196.end L822 L1106.end
  constraint symmetric L192.start L822 L1104.start
  constraint symmetric L184.end L822 L1264.end
  constraint symmetric L191.start L822 L1104.end
  constraint symmetric L202.end L822 L1115.end
  constraint symmetric L203.end L822 L1408.end
  constraint symmetric L186.start L822 L1290.end
  constraint symmetric L186.end L822 L1451.end
  constraint symmetric L198.end L822 L1290.start
  constraint symmetric L187.end L822 L1270.end
  constraint symmetric L188.end L822 L1108.end
  constraint symmetric L206.start L822 L1127.end
  constraint symmetric L190.end L822 L1109.start
  constraint symmetric L205.start L822 L1133.end
  constraint symmetric L193.start L822 L1378.start
  constraint symmetric L193.end L822 L1092.start
  constraint symmetric L194.end L822 L1105.end
  constraint symmetric L208.end L822 L1114.start
  constraint symmetric L197.start L822 L1109.end
  constraint symmetric L198.start L822 L1465.start
  constraint symmetric L204.end L822 L1120.start
  constraint symmetric L201.start L822 L1116.start
  constraint symmetric L201.end L822 L1116.end
  constraint symmetric P4 L822 P8
  constraint symmetric L213.start L822 L1092.end
  constraint symmetric L213.end L822 L1130.end
  constraint symmetric L209.end L822 L1401.end
  constraint symmetric L220.start L822 L1169.start
  constraint symmetric L220.end L822 L1173.end
  constraint symmetric L221.end L822 L1169.end
  constraint symmetric L222.end L822 L1180.start
  constraint symmetric P5 L822 P7
  constraint symmetric L226.start L822 L1165.start
  constraint symmetric L226.end L822 L1165.end
  constraint symmetric L227.start L822 L1186.start
  constraint symmetric L228.start L822 L1201.end
  constraint symmetric L230.start L822 L855.start
  constraint symmetric L230.end L822 L834.start
  constraint symmetric L231.start L822 L849.end
  constraint symmetric L232.start L822 L834.end
  constraint symmetric L234.start L822 L881.end
  constraint symmetric L234.end L822 L880.start
  constraint symmetric L235.start L822 L881.start
  constraint symmetric L236.start L822 L880.end
  constraint symmetric L238.start L822 L1327.end
  constraint symmetric L238.end L822 L1373.end
  constraint symmetric L239.start L822 L1327.start
  constraint symmetric L240.start L822 L1389.end
  constraint symmetric L242.start L822 L1090.end
  constraint symmetric L242.end L822 L1371.end
  constraint symmetric L243.start L822 L1090.start
  constraint symmetric L244.start L822 L1397.start
  constraint symmetric L246.start L822 L1111.end
  constraint symmetric L246.end L822 L1313.end
  constraint symmetric L247.start L822 L1111.start
  constraint symmetric L248.start L822 L1375.end
  constraint symmetric L250.start L822 L1297.start
  constraint symmetric L250.end L822 L1269.start
  constraint symmetric L251.start L822 L1280.end
  constraint symmetric L252.start L822 L1269.end
  constraint symmetric L254.start L822 L1254.end
  constraint symmetric L254.end L822 L1287.end
  constraint symmetric L255.start L822 L1254.start
  constraint symmetric L256.start L822 L1289.end
  constraint symmetric L258.start L822 L1263.end
  constraint symmetric L258.end L822 L1282.end
  constraint symmetric L259.start L822 L1263.start
  constraint symmetric L260.start L822 L1467.start
  constraint symmetric L262.start L822 L1036.end
  constraint symmetric L262.end L822 L1590.start
  constraint symmetric L263.start L822 L1036.start
  constraint symmetric L264.start L822 L1049.start
  constraint symmetric L266.start L822 L1032.end
  constraint symmetric L266.end L822 L1033.start
  constraint symmetric L267.start L822 L1032.start
  constraint symmetric L268.start L822 L1033.end
  constraint symmetric L270.start L822 L992.start
  constraint symmetric L270.end L822 L992.end
  constraint symmetric L271.start L822 L995.end
  constraint symmetric L272.start L822 L995.start
  constraint symmetric L274.start L822 L1001.end
  constraint symmetric L274.end L822 L994.start
  constraint symmetric L275.start L822 L991.end
  constraint symmetric L276.start L822 L991.start
  constraint symmetric L278.start L822 L990.end
  constraint symmetric L278.end L822 L993.start
  constraint symmetric L279.start L822 L990.start
  constraint symmetric L280.start L822 L993.end
  constraint symmetric L282.start L822 L1046.end
  constraint symmetric L282.end L822 L1067.start
  constraint symmetric L283.start L822 L1046.start
  constraint symmetric L284.start L822 L1061.start
  constraint symmetric L286.start L822 L1581.start
  constraint symmetric L286.end L822 L1068.start
  constraint symmetric L287.start L822 L1055.end
  constraint symmetric L288.start L822 L1055.start
  constraint symmetric L290.start L822 L927.start
  constraint symmetric L290.end L822 L927.end
  constraint symmetric L291.start L822 L1170.end
  constraint symmetric L292.start L822 L1019.end
  constraint symmetric L294.start L822 L919.start
  constraint symmetric L294.end L822 L919.end
  constraint symmetric L295.start L822 L934.end
  constraint symmetric L296.start L822 L934.start
  constraint symmetric L298.start L822 L1069.start
  constraint symmetric L298.end L822 L1069.end
  constraint symmetric L299.start L822 L1004.end
  constraint symmetric L300.start L822 L1004.start
  constraint symmetric L302.start L822 L1239.start
  constraint symmetric L302.end L822 L1239.end
  constraint symmetric L303.start L822 L1233.end
  constraint symmetric L304.start L822 L1233.start
  constraint symmetric L306.start L822 L1232.end
  constraint symmetric L306.end L822 L1078.start
  constraint symmetric L307.start L822 L1232.start
  constraint symmetric L308.start L822 L1078.end
  constraint symmetric L310.start L822 L1502.start
  constraint symmetric L310.end L822 L1492.start
  constraint symmetric L311.start L822 L1447.end
  constraint symmetric L312.start L822 L1447.start
  constraint symmetric L314.start L822 L1537.start
  constraint symmetric L314.end L822 L1466.start
  constraint symmetric L315.start L822 L1312.end
  constraint symmetric L316.start L822 L1312.start
  constraint symmetric L318.start L822 L1348.end
  constraint symmetric L318.end L822 L1341.start
  constraint symmetric L319.start L822 L1348.start
  constraint symmetric L320.start L822 L1341.end
  constraint symmetric L322.start L822 L1309.end
  constraint symmetric L322.end L822 L1321.end
  constraint symmetric L323.start L822 L1309.start
  constraint symmetric L324.start L822 L1382.end
  constraint symmetric L326.start L822 L1509.end
  constraint symmetric L326.end L822 L1329.start
  constraint symmetric L327.start L822 L1302.end
  constraint symmetric L328.start L822 L1302.start
  constraint symmetric L330.start L822 L1457.start
  constraint symmetric L330.end L822 L1457.end
  constraint symmetric L331.start L822 L1349.end
  constraint symmetric L332.start L822 L1349.start
  constraint symmetric L334.start L822 L1497.end
  constraint symmetric L334.end L822 L1318.start
  constraint symmetric L335.start L822 L1497.start
  constraint symmetric L336.start L822 L1318.end
  constraint symmetric L338.start L822 L1338.start
  constraint symmetric L338.end L822 L1338.end
  constraint symmetric L339.start L822 L1499.end
  constraint symmetric L340.start L822 L1499.start
  constraint symmetric L342.start L822 L1156.start
  constraint symmetric L342.end L822 L1141.start
  constraint symmetric L343.start L822 L1150.end
  constraint symmetric L344.start L822 L1141.end
  constraint symmetric L346.start L822 L923.end
  constraint symmetric L346.end L822 L907.start
  constraint symmetric L347.start L822 L909.end
  constraint symmetric L348.start L822 L907.end
  constraint symmetric L350.start L822 L837.end
  constraint symmetric L350.end L822 L835.start
  constraint symmetric L351.start L822 L837.start
  constraint symmetric L352.start L822 L835.end
  constraint symmetric L354.start L822 L946.start
  constraint symmetric L354.end L822 L946.end
  constraint symmetric L355.start L822 L1557.end
  constraint symmetric L356.start L822 L1553.end
  constraint symmetric L358.start L822 L1394.end
  constraint symmetric L358.end L822 L1096.start
  constraint symmetric L359.start L822 L1347.end
  constraint symmetric L360.start L822 L1096.end
  constraint symmetric L362.start L822 L1403.start
  constraint symmetric L362.end L822 L1372.start
  constraint symmetric L363.start L822 L1381.end
  constraint symmetric L364.start L822 L1372.end
  constraint symmetric L366.start L822 L1386.start
  constraint symmetric L366.end L822 L1112.start
  constraint symmetric L367.start L822 L1361.end
  constraint symmetric L368.start L822 L1112.end
  constraint symmetric L370.start L822 L1296.end
  constraint symmetric L370.end L822 L1261.start
  constraint symmetric L371.start L822 L1296.start
  constraint symmetric L372.start L822 L1261.end
  constraint symmetric L374.start L822 L1262.start
  constraint symmetric L374.end L822 L1262.end
  constraint symmetric L375.start L822 L1278.end
  constraint symmetric L376.start L822 L1278.start
  constraint symmetric L378.start L822 L1279.start
  constraint symmetric L378.end L822 L1279.end
  constraint symmetric L379.start L822 L1255.end
  constraint symmetric L380.start L822 L1255.start
  constraint symmetric L382.start L822 L1035.start
  constraint symmetric L382.end L822 L1035.end
  constraint symmetric L383.start L822 L1063.start
  constraint symmetric L384.start L822 L1589.end
  constraint symmetric L386.start L822 L1056.start
  constraint symmetric L386.end L822 L1056.end
  constraint symmetric L387.start L822 L1065.start
  constraint symmetric L388.start L822 L1582.end
  constraint symmetric L390.start L822 L1011.end
  constraint symmetric L390.end L822 L1013.end
  constraint symmetric L391.start L822 L989.end
  constraint symmetric L392.start L822 L989.start
  constraint symmetric L394.start L822 L1003.end
  constraint symmetric L394.end L822 L974.start
  constraint symmetric L395.start L822 L1003.start
  constraint symmetric L396.start L822 L974.end
  constraint symmetric L398.start L822 L1022.start
  constraint symmetric L398.end L822 L1016.start
  constraint symmetric L399.start L822 L983.end
  constraint symmetric L400.start L822 L983.start
  constraint symmetric L402.start L822 L1059.end
  constraint symmetric L402.end L822 L1585.end
  constraint symmetric L403.start L822 L1045.end
  constraint symmetric L404.start L822 L1045.start
  constraint symmetric L406.start L822 L1573.end
  constraint symmetric L406.end L822 L1040.start
  constraint symmetric L407.start L822 L1573.start
  constraint symmetric L408.start L822 L1040.end
  constraint symmetric L410.start L822 L910.end
  constraint symmetric L410.end L822 L1167.start
  constraint symmetric L411.start L822 L910.start
  constraint symmetric L412.start L822 L1152.start
  constraint symmetric L414.start L822 L914.end
  constraint symmetric L414.end L822 L916.end
  constraint symmetric L415.start L822 L914.start
  constraint symmetric L416.start L822 L921.end
  constraint symmetric L418.start L822 L1217.end
  constraint symmetric L418.end L822 L1212.start
  constraint symmetric L419.start L822 L1002.end
  constraint symmetric L420.start L822 L1002.start
  constraint symmetric L422.start L822 L1085.end
  constraint symmetric L422.end L822 L1088.start
  constraint symmetric L423.start L822 L1085.start
  constraint symmetric L424.start L822 L1088.end
  constraint symmetric L426.start L822 L1266.end
  constraint symmetric L426.end L822 L1288.start
  constraint symmetric L427.start L822 L1086.end
  constraint symmetric L428.start L822 L1086.start
  constraint symmetric L430.start L822 L1350.end
  constraint symmetric L430.end L822 L1342.start
  constraint symmetric L431.start L822 L1304.end
  constraint symmetric L432.start L822 L1304.start
  constraint symmetric L434.start L822 L1512.end
  constraint symmetric L434.end L822 L1531.start
  constraint symmetric L435.start L822 L1353.end
  constraint symmetric L436.start L822 L1353.start
  constraint symmetric L438.start L822 L1395.end
  constraint symmetric L438.end L822 L1370.start
  constraint symmetric L439.start L822 L1395.start
  constraint symmetric L440.start L822 L1370.end
  constraint symmetric L442.start L822 L1310.start
  constraint symmetric L442.end L822 L1310.end
  constraint symmetric L443.start L822 L1334.start
  constraint symmetric L444.start L822 L1357.end
  constraint symmetric L446.start L822 L1314.end
  constraint symmetric L446.end L822 L1491.start
  constraint symmetric L447.start L822 L1314.start
  constraint symmetric L448.start L822 L1491.end
  constraint symmetric L450.start L822 L1315.start
  constraint symmetric L450.end L822 L1315.end
  constraint symmetric L451.start L822 L1322.end
  constraint symmetric L452.start L822 L1322.start
  constraint symmetric L454.start L822 L1305.end
  constraint symmetric L454.end L822 L1355.start
  constraint symmetric L455.start L822 L1305.start
  constraint symmetric L456.start L822 L1317.start
  constraint symmetric L458.start L822 L1307.end
  constraint symmetric L458.end L822 L1298.start
  constraint symmetric L459.start L822 L1307.start
  constraint symmetric L460.start L822 L1298.end
  constraint symmetric L462.start L822 L931.end
  constraint symmetric L462.end L822 L920.start
  constraint symmetric L463.start L822 L918.end
  constraint symmetric L464.start L822 L918.start
  constraint symmetric L466.start L822 L839.start
  constraint symmetric L466.end L822 L839.end
  constraint symmetric L467.start L822 L840.end
  constraint symmetric L468.start L822 L840.start
  constraint symmetric L470.start L822 L949.end
  constraint symmetric L470.end L822 L958.end
  constraint symmetric L471.start L822 L949.start
  constraint symmetric L472.start L822 L961.end
  constraint symmetric L474.start L822 L824.start
  constraint symmetric L474.end L822 L824.end
  constraint symmetric L475.start L822 L869.start
  constraint symmetric L476.start L822 L866.end
  constraint symmetric L478.start L822 L1484.end
  constraint symmetric L478.end L822 L1445.start
  constraint symmetric L479.start L822 L1455.end
  constraint symmetric L480.start L822 L1445.end
  constraint symmetric L482.start L822 L1323.start
  constraint symmetric L482.end L822 L1323.end
  constraint symmetric L483.start L822 L1461.start
  constraint symmetric L484.start L822 L1437.end
  constraint symmetric L486.start L822 L1500.end
  constraint symmetric L486.end L822 L1483.start
  constraint symmetric L487.start L822 L1473.end
  constraint symmetric L488.start L822 L1473.start
  constraint symmetric L490.start L822 L1214.end
  constraint symmetric L490.end L822 L1286.start
  constraint symmetric L491.start L822 L1214.start
  constraint symmetric L492.start L822 L1253.start
  constraint symmetric L494.start L822 L1272.start
  constraint symmetric L494.end L822 L1272.end
  constraint symmetric L495.start L822 L1281.end
  constraint symmetric L496.start L822 L1281.start
  constraint symmetric L498.start L822 L1213.start
  constraint symmetric L498.end L822 L1213.end
  constraint symmetric L499.start L822 L1274.end
  constraint symmetric L500.start L822 L1265.end
  constraint symmetric L502.start L822 L1038.start